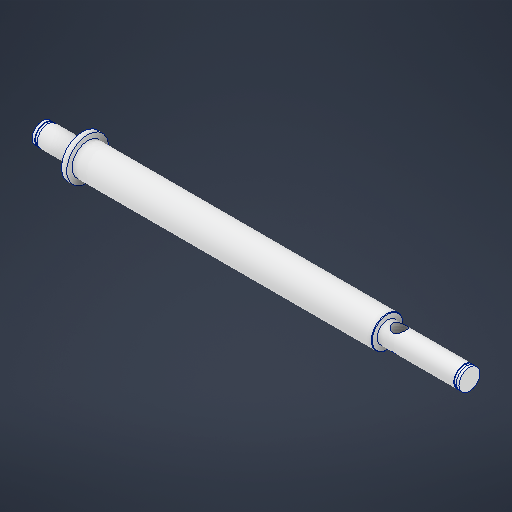
# Autodesk Inventor part: DribblerWelle
Saved by Autodesk Inventor 2025.2 (Build 292293000, 293)
## iProperties
Created: 2024-11-27
Part Number: DribblerWelle
Material: Generisch
Document SubType Name: Modeling
Designer: Fabian
Density: 1 g/cm^3
Appearance: Aluminium - flach
Author: Fabian
Autodesk Inventor part; units mm, degrees
ref_plane "YZ Plane" through (0, 0, 0) normal (1, 0, 0) x (0, 1, 0)
ref_plane "XZ Plane" through (0, 0, 0) normal (0, 1, 0) x (-1, 0, 0)
ref_plane "XY Plane" through (0, 0, 0) normal (0, 0, 1) x (1, 0, 0)
sketch "Skizze1" plane through (0, 0, 0) normal (0, 0, 1) x (1, 0, 0)
  line L0 (0, 0) -> (-39.55, 0)
  line L1 (-39.55, 0) -> (-39.55, 2)
  line L2 (-39.55, 2) -> (-33.35, 2)
  line L3 (-33.35, 2) -> (-33.35, 2.5)
  line L4 (-33.35, 2.5) -> (-33.05, 2.5)
  line L5 (-33.05, 2.5) -> (-33.05, 4)
  line L6 (-33.05, 4) -> (-32.05, 4)
  line L7 (-32.05, 4) -> (-32.05, 3)
  line L8 (0, 0) -> (0, 3) construction
  line L9 (0, 3) -> (-32.05, 3)
  line L10 (0, 0) -> (39.55, 0)
  line L11 (39.55, 0) -> (39.55, 2)
  line L12 (39.55, 2) -> (33.3, 2)
  line L13 (33.3, 2) -> (33.05, 2)
  line L14 (33.05, 2) -> (25.05, 2)
  line L15 (0, 3) -> (25.05, 3)
  line L16 (25.05, 3) -> (25.05, 2)
  line L17 (-39.55, 2) -> (-39.65, 2)
  line L18 (-39.65, 2) -> (-39.65, 1.85)
  line L19 (-39.65, 1.85) -> (-40.15, 1.85)
  line L20 (-40.15, 1.85) -> (-40.15, 2)
  line L21 (-40.15, 2) -> (-40.65, 2)
  line L22 (-40.65, 2) -> (-40.65, 0)
  line L23 (-40.65, 0) -> (-39.55, 0)
  line L24 (39.55, 2) -> (39.65, 2)
  line L25 (39.65, 2) -> (39.65, 1.85)
  line L26 (39.65, 1.85) -> (40.15, 1.85)
  line L27 (40.15, 1.85) -> (40.15, 2)
  line L28 (40.15, 2) -> (40.65, 2)
  line L29 (40.65, 2) -> (40.65, 0)
  line L30 (40.65, 0) -> (39.55, 0)
  dimension "d0" = 39.55
  dimension "d1" = 2
  dimension "d2" = 6.2
  dimension "d3" = 0.5
  dimension "d4" = 0.3
  dimension "d5" = 1.5
  dimension "d6" = 1
  dimension "d7" = 3
  dimension "d8" = 32.05
  dimension "d9" = 39.55
  dimension "d10" = 2
  dimension "d13" = 0.25
  dimension "d14" = 8
  dimension "d16" = 25.05
  dimension "d17" = 0.1
  dimension "d18" = 0.15
  dimension "d19" = 0.5
  dimension "d20" = 0.5
  dimension "d21" = 0.1
  dimension "d22" = 0.15
  dimension "d23" = 0.5
  dimension "d24" = 0.5
  constraints: 62 end point, 14 perpendicular, 10 horizontal, 4 vertical, 3 point on line, 1 parallel
  measures "d0" distance of L0.start L0.end
  measures "d1" distance of L0.end L1.end
  measures "d2" distance of L1.end L2.end
  measures "d3" distance of L2.end L3.end
  measures "d4" distance of L3.end L4.end
  measures "d5" distance of L4.end L5.end
  measures "d6" distance of L5.end L6.end
  measures "d7" distance of L0.start L8.end
  measures "d8" distance of L8.end L7.end
  measures "d9" distance of L0.start L10.end
  measures "d10" distance of L10.end L11.end
  measures "d13" distance of L12.end L13.end
  measures "d14" distance of L13.end L14.end
  measures "d16" distance of L8.end L15.end
  measures "d17" distance of L1.end L17.end
  measures "d18" distance of L17.end L18.end
  measures "d19" distance of L18.end L19.end
  measures "d20" distance of L20.end L21.end
  measures "d21" distance of L11.end L24.end
  measures "d22" distance of L24.end L25.end
  measures "d23" distance of L25.end L26.end
  measures "d24" distance of L27.end L28.end
revolve "Umdrehung1" add sketch "Skizze1" angle 360 about axis through (0, 0, 0) along (-1, 0, 0)
sketch "Skizze2" plane through (0, 0, 0) normal (0, 1, 0) x (-1, 0, 0)
  line L0 (-25.05, -3) -> (-25.05, 3) projected
  line L1 (-25.05, 0) -> (-27.3, 0)
  point P0 (0, 0)
  dimension "d26" = 2.25
  constraints: 2 end point, 1 coincident, 1 horizontal, 1 midpoint
  measures "d26" distance of L1.start L1.end
hole "Bohrung1" at (27.3, 0, 0) direction (0, -1, 0) diameter 2.459 depth 8.8 thread size "M3x0.5" class "6H" standard "ISO Metric profile"
hole "Bohrung2" at (27.3, 0, 0) direction (0, 1, 0) diameter 2.459 depth 8.8 thread size "M3x0.5" class "6H" standard "ISO Metric profile"
chamfer "Fasen1" distance 0.1 angle 45 1 edges at (25.05, -3, 0)
